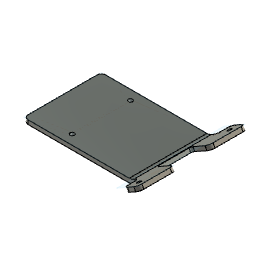
Elegoo_camera_v1 (Autodesk Fusion 360 design; units mm, degrees)
Autodesk Fusion 360 part; units mm, degrees
sketch "Sketch1" plane through (0, 0, 0) normal (0, 1, 0) x (1, 0, 0)
  line L0 (25, -0.95) -> (-25, -0.95)
  line L1 (-25, -0.95) -> (-25, 0.95)
  line L2 (-25, 0.95) -> (25, 0.95)
  line L3 (25, 0.95) -> (25, -0.95)
  line L4 (25, -0.95) -> (-25, 0.95) construction
  line L5 (-25, -0.95) -> (25, 0.95) construction
  line L6 (25, -0.95) -> (34.7861, -6.6)
  line L7 (25, -0.95) -> (36.3, -0.95) construction
  line L8 (34.7861, -6.6) -> (35.7361, -4.9546)
  line L9 (35.7361, -4.9546) -> (25, 0.95)
  dimension "d1" = 50
  dimension "d2" = 1.9
  dimension "d3" = 30
  dimension "d4" = 11.3
  dimension "d5" = 1.9
  constraint horizontal L0
  constraint perpendicular L0 L1
  constraint parallel L0 L2
  constraint parallel L1 L3
  constraint coincident L4 origin
  constraint coincident L5 origin
  constraint horizontal L7
  constraint perpendicular L6 L8
  measures "d1" distance of L1.end L2.end
  measures "d2" distance of L0.end L1.end
  measures "d3" angle of L6 L7
  measures "d4" distance of L0.start L6.end
  measures "d5" distance of L6.end L8.end
extrude "Extrude1" add sketch "Sketch1" along normal blind 50
sketch "Sketch2" plane through (5.8386, 0, -10.1128) normal (-0.5, 0, 0.866025) x (0, -1, 0)
  line L0 (0, 22.1256) -> (0, 33.4256)
  line L1 (0, 33.4256) -> (-50, 33.4256)
  line L2 (-50, 33.4256) -> (-50, 22.1256)
  line L3 (-50, 22.1256) -> (0, 22.1256)
  line L4 (-17, 30) -> (-33, 30)
  line L5 (-33, 30) -> (-33, 36.8513)
  line L6 (-33, 36.8513) -> (-17, 36.8513)
  line L7 (-17, 36.8513) -> (-17, 30)
  line L8 (-17, 30) -> (-33, 36.8513) construction
  line L9 (-33, 30) -> (-17, 36.8513) construction
  point P0 (-25, 33.4256)
  dimension "d8" = 16
  constraint horizontal L4
  constraint perpendicular L4 L5
  constraint parallel L4 L6
  constraint parallel L5 L7
  constraint coincident L8 P0
  constraint coincident L9 P0
  constraint midpoint L1 P0
  measures "d8" distance of L5.end L6.end
extrude "Extrude2" cut sketch "Sketch2" against normal blind 11 contours L1 L4 L5 L7
sketch "Sketch3" plane through (5.8386, 0, -10.1128) normal (-0.5, 0, 0.866025) x (0, -1, 0)
  line L0 (-17, 33.4256) -> (-17, 30)
  line L1 (-17, 30) -> (-33, 30)
  line L2 (-33, 30) -> (-33, 33.4256)
  line L3 (-33, 33.4256) -> (-50, 33.4256)
  line L4 (-50, 33.4256) -> (-50, 22.1256)
  line L5 (-50, 22.1256) -> (0, 22.1256)
  line L6 (0, 22.1256) -> (0, 33.4256)
  line L7 (0, 33.4256) -> (-17, 33.4256)
sketch "Sketch4" plane through (0, 0, 0.95) normal (0, 0, 1) x (-1, 0, 0)
  line L0 (25, 0) -> (-25, 0)
  line L1 (-25, 0) -> (-25, -50)
  line L2 (-25, -50) -> (25, -50)
  line L3 (25, -50) -> (25, 0)
  line L4 (-25, -50) -> (25, -50)
  line L5 (25, -50) -> (25, -43)
  line L6 (25, -43) -> (-25, -43)
  line L7 (-25, -43) -> (-25, -50)
  dimension "d11" = 7
  constraint horizontal L4
  constraint vertical L5
  constraint horizontal L6
  constraint vertical L7
  constraint coincident L1.end L2.start
  measures "d11" distance of L1.end L6.end
sketch "Sketch5" plane through (5.8386, 0, -10.1128) normal (-0.5, 0, 0.866025) x (0, -1, 0)
  line L0 (-43, 22) -> (-50, 22)
  line L1 (-50, 22) -> (-50, 26)
  line L2 (-50, 26) -> (-43, 26)
  line L3 (-43, 26) -> (-43, 22)
  dimension "d12" = 4
  constraint horizontal L0
  constraint vertical L1
  constraint horizontal L2
  constraint vertical L3
  measures "d12" distance of L0.start L2.end
extrude "Extrude3" cut sketch "Sketch5" against normal blind 3.276
extrude "Extrude4" cut sketch "Sketch4" against normal blind 5 contours L1 L2 L3 L4 L5 L6 L7
extrude "Extrude5" cut 1 faces at (25.2408, 50, -0.268) along direction (0, -1, 0) blind 7
sketch "Sketch6" plane through (0, 0, 0.95) normal (0, 0, 1) x (-1, 0, 0)
  line L0 (-25, -43) -> (25, -43)
  line L1 (25, -43) -> (25, 0)
  line L2 (25, 0) -> (-25, 0)
  line L3 (-25, 0) -> (-25, -43)
  line L4 (25, 0) -> (-25, 0)
  line L5 (-25, 0) -> (-25, -7)
  line L6 (-25, -7) -> (25, -7)
  line L7 (25, -7) -> (25, 0)
  dimension "d19" = 7
  constraint horizontal L4
  constraint vertical L5
  constraint horizontal L6
  constraint vertical L7
  constraint coincident L1.end L2.start
  measures "d19" distance of L1.end L6.end
sketch "Sketch7" plane through (5.8386, 0, -10.1128) normal (-0.5, 0, 0.866025) x (0, -1, 0)
  line L0 (0, 22) -> (-7, 22)
  line L1 (-7, 22) -> (-7, 26)
  line L2 (-7, 26) -> (0, 26)
  line L3 (0, 26) -> (0, 22)
  constraint horizontal L0
  constraint vertical L1
  constraint horizontal L2
  constraint vertical L3
extrude "Extrude6" cut sketch "Sketch6" against normal blind 3 contours L1 L2 L3 L4 L5 L6 L7
extrude "Extrude7" cut sketch "Sketch7" against normal blind 5
extrude "Extrude8" cut 1 faces at (25.2408, 0, -0.268) along direction (0, 1, 0) blind 7
sketch "Sketch8" plane through (0, 0, 0.95) normal (0, 0, 1) x (-1, 0, 0)
  line L0 (25, -7) -> (-25, -7)
  line L1 (-25, -7) -> (-25, -43)
  line L2 (-25, -43) -> (25, -43)
  line L3 (25, -43) -> (25, -7)
sketch "Sketch9" plane through (0, 0, 0.95) normal (0, 0, 1) x (-1, 0, 0)
  circle A0 centre (7, -11.5) radius 1
  line L0 (25, -43) -> (25, -7)
  circle A1 centre (7, -38.5) radius 1
  line L1 (25, -7) -> (-25, -7)
  dimension "d27" = 2
  dimension "d28" = 18
  dimension "d29" = 18
  dimension "d30" = 27
  dimension "d31" = 4.5
  measures "d27" diameter of A0
  measures "d28" distance of A0.centre L0
  measures "d29" distance of L0 A1.centre
  measures "d30" distance of A0.centre A1.centre
  measures "d31" distance of A0.centre L1
extrude "Extrude9" cut sketch "Sketch9" against normal blind 3
sketch "Sketch10" plane through (5.8386, 0, -10.1128) normal (-0.5, 0, 0.866025) x (0, -1, 0)
  circle A0 centre (-4, 29.6756) radius 1
  circle A1 centre (-46, 29.6756) radius 1
  line L0 (0, 33.4256) -> (-17, 33.4256)
  dimension "d34" = 2
  dimension "d35" = 2
  dimension "d36" = 42
  dimension "d37" = 3.75
  measures "d34" diameter of A0
  measures "d35" diameter of A1
  measures "d36" distance of A0.centre A1.centre
  measures "d37" distance of A0.centre L0
extrude "Extrude10" cut sketch "Sketch10" against normal blind 6
fillet "Fillet1" radius 2 8 edges at (28.7917, 50, 2.1313) (35.2611, 50, 5.7773) (-25, 43, 0) (-25, 7, 0) (28.7917, 0, 2.1313) (35.2611, 0, 5.7773) (35.2611, 33, 5.7773) (35.2611, 17, 5.7773)
sketch "Sketch11" plane through (5.8386, 0, -10.1128) normal (-0.5, 0, 0.866025) x (0, -1, 0)
  line L0 (-33, 30) -> (-17, 30)
  line L1 (-17, 30) -> (-17, 24)
  line L2 (-17, 24) -> (-33, 24)
  line L3 (-33, 24) -> (-33, 30)
  constraint horizontal L0
  constraint vertical L1
  constraint horizontal L2
  constraint vertical L3
extrude "Extrude11" cut sketch "Sketch11" against normal blind 7.5
fillet "Fillet2" radius 4 1 edges at (25, 25, 0.95)
fillet "Fillet3" radius 5.75 1 edges at (25, 25, -0.95)
fillet "Fillet4" radius 1 2 edges at (27.0493, 33, 1.1493) (27.0493, 17, 1.1493)
fillet "Fillet5" radius 1.5 2 edges at (28.7917, 43, 2.1313) (28.7917, 7, 2.1313)
